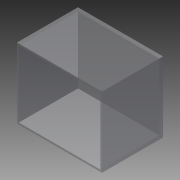
# Autodesk Inventor part: Box Bottom
Saved by Autodesk Inventor 2013 (Build 170138000, 138)
## iProperties
Created: 2013-06-27
Part Number: Box Bottom
Material: Generic
Document SubType Name: Modeling
Designer: Kyle
Density: 1 g/cm^3
Author: Kyle
Autodesk Inventor part; units mm, degrees
ref_plane "YZ Plane" through (0, 0, 0) normal (1, 0, 0) x (0, 1, 0)
ref_plane "XZ Plane" through (0, 0, 0) normal (0, 1, 0) x (-1, 0, 0)
ref_plane "XY Plane" through (0, 0, 0) normal (0, 0, 1) x (1, 0, 0)
sketch "Sketch1" plane through (0, 0, 0) normal (0, 0, 1) x (1, 0, 0)
  line L0 (0, 0) -> (58.42, 0)
  line L1 (58.42, 0) -> (58.42, -48.26)
  line L2 (58.42, -48.26) -> (0, -48.26)
  line L3 (0, -48.26) -> (0, 0)
  dimension "d0" = 58.42
  dimension "d1" = 48.26
  constraints: 8 end point, 2 parallel, 1 horizontal, 1 perpendicular
  measures "d0" distance of L0.start L0.end
  measures "d1" distance of L2.end L0.start
extrude "Extrusion1" add sketch "Sketch1" along normal blind 1.27
sketch "Sketch2" plane through (0, 0, 1.27) normal (0, 0, 1) x (1, 0, 0)
  line L0 (58.42, 0) -> (0, 0) projected
  line L1 (0, 0) -> (0, -48.26) projected
  line L2 (0, -48.26) -> (58.42, -48.26) projected
  line L3 (58.42, -48.26) -> (58.42, 0) projected
  line L4 (1.27, -1.27) -> (57.15, -1.27)
  line L5 (57.15, -1.27) -> (57.15, -46.99)
  line L6 (57.15, -46.99) -> (1.27, -46.99)
  line L7 (1.27, -46.99) -> (1.27, -1.27)
  dimension "d4" = 1.27
  dimension "d5" = 1.27
  dimension "d6" = 1.27
  dimension "d7" = 1.27
  constraints: 8 end point, 2 parallel, 1 horizontal, 1 perpendicular
  measures "d4" distance between parallel lines of L0 L4
  measures "d5" distance between parallel lines of L3 L5
  measures "d6" distance between parallel lines of L6 L2
  measures "d7" distance between parallel lines of L1 L7
extrude "Extrusion2" add sketch "Sketch2" along normal blind 40.64
body "Solid1"
